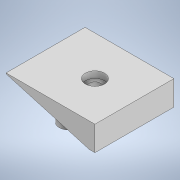
# Autodesk Inventor part: aruco_attachment_v1
Saved by Autodesk Inventor 2022 (Build 260153000, 153)
## iProperties
Created: 2022-09-07
Part Number: aruco_attachment_v1
Material: Generic
Document SubType Name: Modeling
Designer: kylem
Density: 1 g/cm^3
Appearance: Default
Author: kylem
Autodesk Inventor part; units mm, degrees
ref_plane "YZ Plane" through (0, 0, 0) normal (1, 0, 0) x (0, 1, 0)
ref_plane "XZ Plane" through (0, 0, 0) normal (0, 1, 0) x (-1, 0, 0)
ref_plane "XY Plane" through (0, 0, 0) normal (0, 0, 1) x (1, 0, 0)
sketch "Sketch1" plane through (0, 0, 0) normal (0, 1, 0) x (-1, 0, 0)
  line L0 (0, 0) -> (27, 0)
  line L1 (27, 0) -> (27, -24)
  line L2 (27, -24) -> (0, -24)
  line L3 (0, -24) -> (0, 0)
  dimension "d0" = 27
  dimension "d1" = 24
  constraints: 8 end point, 2 parallel, 1 horizontal, 1 perpendicular
  measures "d0" distance of L1.end L2.end
  measures "d1" distance of L0.end L1.end
extrude "Extrusion1" add sketch "Sketch1" along normal blind 8
sketch "Sketch2" plane through (0, 0, -24) normal (0, 0, -1) x (-1, 0, 0)
  line L0 (0, 0) -> (27, 0) projected
  line L1 (0, 0) -> (46.1678, 13.2384)
  line L2 (0, 0) -> (48.0283, 0) construction
  line L3 (0, 8) -> (27, 8) projected
  line L4 (27, 0) -> (27, 8) projected
  line L5 (0, 8) -> (27, 8)
  line L6 (27, 8) -> (27, 0)
  line L7 (27, 0) -> (0, 0)
  line L8 (0, 0) -> (0, 8)
  point P0 (27, 7.7421)
  dimension "d4" = 16
  constraints: 12 end point, 2 horizontal, 2 parallel, 1 equal length, 1 perpendicular
  measures "d4" angle of L2 L1
extrude "Extrusion2" cut sketch "Sketch2" against normal blind 30 contours L1 L4 L0
ref_plane "Work Plane1" through (0, 0, 0) normal (0, -1, 0) x (1, 0, 0)
sketch "Sketch3" plane through (0, 0, 0) normal (0, -1, 0) x (1, 0, 0)
  line L0 (0, 0) -> (0, -24) projected
  line L1 (0, -12) -> (-4, -12)
  circle A0 centre (-4, -12) radius 2.85
  line L2 (-4, -12) -> (-20, -12)
  line L3 (-12, -12) -> (-12, -20)
  line L4 (-12, -20) -> (-12, -4)
  circle A1 centre (-12, -20) radius 2.85
  circle A2 centre (-20, -12) radius 2.85
  circle A3 centre (-12, -4) radius 2.85
  dimension "d8" = 4
  dimension "d9" = 5.7
  dimension "d10" = 16
  dimension "d11" = 8
  dimension "d12" = 16
  dimension "d13" = 5.7
  dimension "d14" = 5.7
  dimension "d15" = 5.7
  constraints: 8 end point, 4 centre point, 4 coincident, 2 horizontal, 2 midpoint, 1 point on line, 1 vertical
  measures "d8" distance of L1.start L1.end
  measures "d9" diameter of A0
  measures "d10" distance of L2.start L2.end
  measures "d11" distance of L3.start L3.end
  measures "d12" distance of L3.end L4.end
  measures "d13" diameter of A1
  measures "d14" diameter of A2
  measures "d15" diameter of A3
extrude "Extrusion3" add sketch "Sketch3" against normal blind 8
sketch "Sketch4" plane through (-4, 0, -12) normal (0, -1, 0) x (1, 0, 0)
  line L0 (4, 12) -> (4, -12) projected
  line L1 (4, -12) -> (-23.2805, -12)
  line L2 (-23.2805, -12) -> (-23.2805, 12)
  line L3 (-23.2805, 12) -> (4, 12)
  line L4 (4, 12) -> (4, -12)
  constraints: 8 end point, 2 parallel, 1 horizontal, 1 perpendicular
extrude "Extrusion4" cut sketch "Sketch4" against normal blind 0.5
sketch "Sketch5" plane through (0, 8, 0) normal (0, 1, 0) x (1, 0, 0)
  line L0 (0, 0) -> (0, 24) projected
  line L1 (-27, 24) -> (-27, 0) projected
  line L2 (0, 0) -> (-27, 0)
  line L3 (-27, 0) -> (-27, 24)
  line L4 (-27, 24) -> (0, 24)
  line L5 (0, 24) -> (0, 0)
  circle A0 centre (-12, 4) radius 2.85 projected
  circle A1 centre (-12, 20) radius 2.85 projected
  line L6 (-12, 4) -> (-12, 20)
  arc A2 (-1.7437, 13.7412) -> (-1.7437, 10.2588) centre (-4, 12) ccw projected
  circle A3 centre (-20, 12) radius 2.85 projected
  line L7 (-4, 12) -> (-20, 12)
  circle A4 centre (-12, 12) radius 1.65
  dimension "d20" = 3.3
  constraints: 12 end point, 2 horizontal, 2 parallel, 1 centre point, 1 midpoint, 1 perpendicular, 1 vertical
  measures "d20" diameter of A4
extrude "Extrusion5" cut sketch "Sketch5" against normal blind 30 contours A4 L7 L6 | L6 L7 A4 | L7 A4 L6 | L6 A4 L7
sketch "Sketch6" plane through (0, 8, 0) normal (0, 1, 0) x (1, 0, 0)
  circle A0 centre (-12, 12) radius 1.65 projected
  circle A1 centre (-12, 12) radius 2.9
  point P0 (0, 0)
  dimension "d23" = 5.8
  constraints: 1 centre point, 1 coincident
  measures "d23" diameter of A1
extrude "Extrusion6" cut sketch "Sketch6" against normal blind 2
sketch "Sketch7" plane through (0, 8, 0) normal (0, 1, 0) x (1, 0, 0)
  line L0 (0, 24) -> (-27, 24) projected
  line L1 (0, 0) -> (-27, 0)
  line L2 (-27, 0) -> (-27, 24)
  line L3 (-27, 24) -> (0, 24)
  line L4 (0, 24) -> (0, 0)
  circle A0 centre (-12, 12) radius 1.65 projected
  circle A1 centre (-12, 12) radius 2.9
  constraints: 8 end point, 2 parallel, 1 centre point, 1 coincident, 1 horizontal, 1 perpendicular
extrude "Extrusion7" add sketch "Sketch7" along normal blind 4 contours L4 L1 L2 L0
sketch "Sketch8" plane through (0, 12, 0) normal (0, 1, 0) x (1, 0, 0)
  circle A0 centre (-12, 12) radius 2.9 projected
  line L0 (-12, 12) -> (-12, -7.1279)
  line L1 (-27, 0) -> (0, 0) projected
  line L2 (-12, 12) -> (3.3617, 12)
  line L3 (3.3617, 12) -> (3.3617, -5.9927)
  line L4 (3.3617, -5.9927) -> (-12, -5.9927)
  line L5 (-12, -5.9927) -> (-12, 12)
  line L6 (-12, 12) -> (-14, 12)
  line L7 (-14, 12) -> (-14, -1.5388)
  line L8 (-12, 12) -> (-12, 14)
  line L9 (-12, 14) -> (5.1891, 14)
  line L10 (-14, -1.5388) -> (5.1891, -1.5388)
  line L11 (5.1891, -1.5388) -> (5.1891, 14)
  line L12 (5.1891, 14) -> (-14, 14)
  line L13 (-14, 14) -> (-14, -1.5388)
  point P0 (-14, 9.9)
  point P1 (-14, 0)
  point P2 (-12, 0)
  point P3 (-12, -1.5388)
  point P4 (-9.9, 14)
  dimension "d28" = 2
  dimension "d29" = 2
  constraints: 26 end point, 5 perpendicular, 4 parallel, 3 horizontal, 1 vertical
  measures "d28" distance of L0.start L6.end
  measures "d29" distance of L0.start L8.end
extrude "Extrusion8" cut sketch "Sketch8" against normal blind 4 contours L2 L3 L10 L0 A0 | A0 L9 L11 L10 L3 L2 | L0 L1 L7 A0
sketch "Sketch10" plane through (0, 12, 0) normal (0, 1, 0) x (1, 0, 0)
  line L0 (0, 14) -> (0, 0) projected
  line L1 (-27, 24) -> (-27, 0) projected
  line L2 (0, 0) -> (-27, 0)
  line L3 (-27, 0) -> (-27, 24)
  line L4 (-27, 24) -> (0, 24)
  line L5 (0, 24) -> (0, 0)
  constraints: 8 end point, 2 parallel, 1 horizontal, 1 perpendicular
extrude "Extrusion10" cut sketch "Sketch10" against normal blind 4
body "Solid1"
